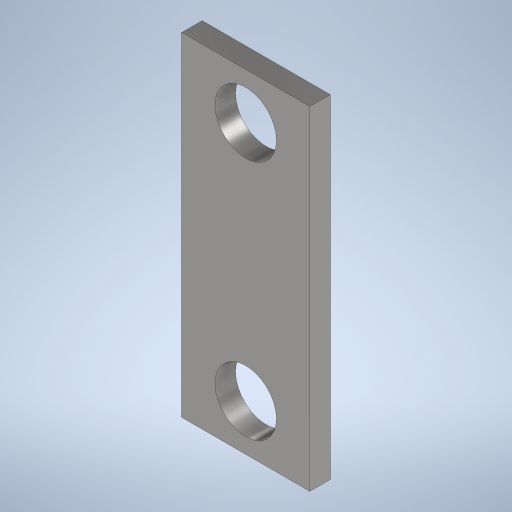
# Autodesk Inventor part: Hook-Extension
Saved by Autodesk Inventor 2023 (Build 270158000, 158)
## iProperties
Created: 2023-12-15
Part Number: Hook-Extension
Material: Steel, Mild
Document SubType Name: Modeling
Designer: User
Density: 7.85 g/cm^3
Appearance: Semi-Polished
Author: User
Autodesk Inventor part; units mm, degrees
ref_plane "YZ Plane" through (0, 0, 0) normal (1, 0, 0) x (0, 1, 0)
ref_plane "XZ Plane" through (0, 0, 0) normal (0, 1, 0) x (-1, 0, 0)
ref_plane "XY Plane" through (0, 0, 0) normal (0, 0, 1) x (1, 0, 0)
sketch "Sketch1" plane through (0, 0, 0) normal (0, 0, 1) x (1, 0, 0)
  line L0 (0, 0) -> (45, 0)
  line L1 (45, 0) -> (45, -65)
  line L2 (45, -65) -> (0, -65)
  line L3 (0, -65) -> (0, 0)
  line L4 (45, 15.0081) -> (45, -81.3497) construction
  line L5 (22.5, 15.0081) -> (22.5, -81.3497) construction
  line L6 (80.9794, 0) -> (-24.1636, 0) construction
  line L7 (80.9794, -9) -> (-24.1636, -9) construction
  circle A0 centre (22.5, -9) radius 6
  line L8 (91.2527, -65) -> (-31.7655, -65) construction
  line L9 (91.2527, -56) -> (-31.7655, -56) construction
  circle A1 centre (22.5, -56) radius 6
  line L10 (0, 6.8812) -> (0, -100.7793) construction
  line L11 (10, 6.8812) -> (10, -100.7793)
  line L12 (35, 15.0081) -> (35, -81.3497)
  point P0 (35, -65)
  point P1 (35, 0)
  point P2 (10, 0)
  point P3 (10, -65)
  dimension "d0" = 45
  dimension "d1" = 65
  dimension "d2" = 22.5
  dimension "d3" = 9
  dimension "d4" = 12
  dimension "d5" = 9
  dimension "d6" = 12
  dimension "d9" = 10
  dimension "d10" = 10
  constraints: 26 end point, 7 parallel, 6 point on line, 3 horizontal, 2 centre point, 1 perpendicular
  measures "d0" distance of L1.end L2.end
  measures "d1" distance of L0.end L1.end
  measures "d2" distance between parallel lines of L4 L5
  measures "d3" distance between parallel lines of L6 L7
  measures "d4" diameter of A0
  measures "d5" distance between parallel lines of L8 L9
  measures "d6" diameter of A1
  measures "d9" distance between parallel lines of L10 L11
  measures "d10" distance between parallel lines of L4 L12
extrude "Extrusion2" add sketch "Sketch1" along normal blind 4 contours L0 L12 L2 L11
body "Solid2"
